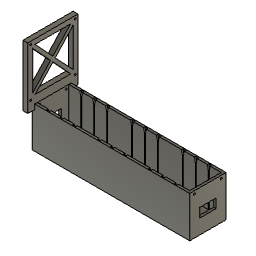
20220629_chipholder (Autodesk Fusion 360 design; units mm, degrees)
Autodesk Fusion 360 part; units mm, degrees
note: some values were not read from the file. Chosen so that the rebuilt part matches the saved one: a direction; which face or edge a step refers to. Set by a fixed rule: which sketch regions a step uses.
sketch "Sketch1" plane through (0, 0, 0) normal (0, 1, 0) x (1, 0, 0)
  line L0 (-25, -80) -> (231.8, -80) construction
  line L1 (0, 0) -> (0, -70.2552)
  line L2 (1.8, -70.2552) -> (1.8, 0)
  line L3 (0, -70.2552) -> (-2, -80)
  line L4 (1.8, -70.2552) -> (3.8, -80)
  line L5 (26.8, 0) -> (26.8, -70.2552)
  line L6 (28.6, -70.2552) -> (28.6, 0)
  line L7 (26.8, -70.2552) -> (24.8, -80)
  line L8 (28.6, -70.2552) -> (30.6, -80)
  line L9 (53.6, -70.2552) -> (53.6, 0)
  line L10 (160.8, 0) -> (160.8, -70.2552)
  line L11 (55.4, -70.2552) -> (55.4, 0)
  line L12 (105.4, 0) -> (105.4, -70.2552)
  line L13 (107.2, -70.2552) -> (107.2, 0)
  line L14 (132.2, 0) -> (132.2, -70.2552)
  line L15 (159, -70.2552) -> (159, 0)
  line L16 (212.6, 0) -> (212.6, -70.2552)
  line L17 (210.8, -70.2552) -> (210.8, 0)
  line L18 (134, 0) -> (134, -70.2552)
  line L19 (53.6, -70.2552) -> (51.6, -80)
  line L20 (55.4, -70.2552) -> (57.4, -80)
  line L21 (105.4, -70.2552) -> (103.4, -80)
  line L22 (132.2, -70.2552) -> (130.2, -80)
  line L23 (210.8, -70.2552) -> (208.8, -80)
  line L24 (212.6, -70.2552) -> (214.6, -80)
  line L25 (107.2, -70.2552) -> (109.2, -80)
  line L26 (134, -70.2552) -> (136, -80)
  line L27 (159, -70.2552) -> (157, -80)
  line L28 (160.8, -70.2552) -> (162.8, -80)
  line L29 (-25, -80) -> (291.2, -80)
  line L30 (291.2, 0) -> (-25, 0)
  line L31 (-25, 0) -> (-25, -80)
  line L32 (237.6, -70.2552) -> (237.6, 0)
  line L33 (239.4, 0) -> (239.4, -70.2552)
  line L34 (266.2, -70.2552) -> (266.2, 0)
  line L35 (264.4, -70.2552) -> (264.3999, 0)
  line L36 (237.6, -70.2552) -> (235.6, -80)
  line L37 (239.4, -70.2552) -> (241.4, -80)
  line L38 (264.4, -70.2552) -> (262.4, -80)
  line L39 (266.2, -70.2552) -> (268.2, -80)
  line L40 (291.2, 0) -> (291.2, -80)
  dimension "d5" = 1.8
  dimension "d6" = 2
  dimension "d7" = 2
  dimension "d8" = 25
  dimension "d9" = 1.8
  dimension "d10" = 2
  dimension "d11" = 2
  dimension "d12" = 25
  dimension "d13" = 1.8
  dimension "d14" = 50
  dimension "d15" = 1.8
  dimension "d16" = 25
  dimension "d17" = 1.8
  dimension "d18" = 25
  dimension "d19" = 1.8
  dimension "d20" = 50
  dimension "d21" = 1.8
  dimension "d22" = 2
  dimension "d23" = 2
  dimension "d24" = 2
  dimension "d25" = 2
  dimension "d26" = 2
  dimension "d27" = 2
  dimension "d28" = 2
  dimension "d29" = 2
  dimension "d30" = 2
  dimension "d31" = 2
  dimension "d89" = 25
  dimension "d90" = 1.8
  dimension "d91" = 25
  dimension "d92" = 1.8
  dimension "d93" = 2
  dimension "d94" = 2
  dimension "d95" = 2
  dimension "d96" = 2
  dimension "d97" = 25
  dimension "d98" = 25
  dimension "d99" = 80
  constraint coincident L0 L3.end
  constraint coincident L0 L4.end
  constraint coincident L0 L7.end
  constraint coincident L0 L8.end
  constraint coincident L0 L19.end
  constraint coincident L0 L20.end
  constraint midpoint L0 L21.end
  constraint coincident L0 L22.end
  constraint coincident L0 L23.end
  constraint coincident L0 L24.end
  constraint coincident L0 L25.end
  constraint coincident L0 L26.end
  constraint coincident L0 L27.end
  constraint coincident L0 L28.end
  constraint horizontal L29
  constraint horizontal L30
  constraint vertical L31
  constraint coincident L30 L32.end
  constraint coincident L30 L33.start
  constraint coincident L29 L36.end
  constraint coincident L29 L37.end
  constraint coincident L29 L38.end
  constraint coincident L29 L39.end
  constraint perpendicular L29 L40
  measures "d5" distance of L1 L2
  measures "d6" distance of L1 L3.end
  measures "d7" distance of L2 L4.end
  measures "d8" distance of L2 L5
  measures "d9" distance of L5 L6
  measures "d10" distance of L5 L7.end
  measures "d11" distance of L6 L8.end
  measures "d12" distance of L6 L9
  measures "d13" distance of L9 L11
  measures "d14" distance of L11 L12
  measures "d15" distance of L12 L13
  measures "d16" distance of L13 L14
  measures "d17" distance of L14 L18
  measures "d18" distance of L15 L18
  measures "d19" distance of L10 L15
  measures "d20" distance of L10 L17
  measures "d21" distance of L16 L17
  measures "d22" distance of L9 L19.end
  measures "d23" distance of L11 L20.end
  measures "d24" distance of L12 L21.end
  measures "d25" distance of L13 L25.end
  measures "d26" distance of L14 L22.end
  measures "d27" distance of L18 L26.end
  measures "d28" distance of L15 L27.end
  measures "d29" distance of L10 L28.end
  measures "d30" distance of L17 L23.end
  measures "d31" distance of L16 L24.end
  measures "d89" distance of L16 L32
  measures "d90" distance of L32 L33
  measures "d91" distance of L33 L35
  measures "d93" distance of L32 L36.end
  measures "d94" distance of L33 L37.end
  measures "d95" distance of L35 L38.end
  measures "d96" distance of L34 L39.end
  measures "d97" distance of L1 L31
  measures "d98" distance of L34 L40
  measures "d99" distance of L29 L30
extrude "Extrude1" add sketch "Sketch1" along normal blind 5 makes body 1
extrude "Extrude2" cut sketch "Sketch1" along normal blind 3 contours L1 L2 L3 L4 L29 L30 | L5 L6 L7 L8 L29 L30 | L9 L11 L19 L20 L29 L30 | L12 L13 L21 L25 L29 L30 | L14 L18 L22 L26 L29 L30 | L10 L15 L27 L28 L29 L30 | L16 L17 L23 L24 L29 L30 bodies 1
sketch "Sketch1 (2)" plane through (0, 0, 0) normal (0, 0, 1) x (1, 0, 0) in component "carrier"
  line L0 (-40.0005, -7.3553) -> (29.9995, -7.3553)
  line L1 (29.9995, -7.3553) -> (29.9995, 62.6447)
  line L2 (-40.0005, 62.6447) -> (-40.0005, -7.3553)
  line L3 (-40.0005, 62.6447) -> (-31.0005, 62.6447)
  line L4 (29.9995, 62.6447) -> (20.9995, 62.6447)
  line L5 (-31.0005, 62.6447) -> (-31.0005, 79.6447)
  line L6 (20.9995, 62.6447) -> (20.9995, 79.6447)
  line L7 (20.9995, 79.6447) -> (44.9995, 79.6447)
  line L8 (44.9995, 79.6447) -> (44.9995, 187.4447)
  line L9 (44.9995, 187.4447) -> (-55.0005, 187.4447)
  line L10 (-55.0005, 187.4447) -> (-55.0005, 79.6447)
  line L11 (-55.0005, 79.6447) -> (-31.0005, 79.6447)
  circle A0 centre (-51.1505, 83.4947) radius 1.95
  circle A1 centre (41.1495, 83.4947) radius 1.95
  circle A2 centre (41.1495, 183.5947) radius 1.95
  circle A3 centre (-51.1505, 183.5947) radius 1.95
  line L12 (75.2881, -7.3553) -> (70.2881, -7.3553)
  dimension "d18_1" = 70
  dimension "d23_1" = 9
  dimension "d24_1_1" = 9
  dimension "d25_1_1" = 70
  dimension "d26_1_1" = 52
  dimension "d27_1_1" = 17
  dimension "d28_1" = 17
  dimension "d29_1_1" = 70
  dimension "d47" = 107.8
  dimension "d48" = 100
  dimension "d49" = 3.9
  dimension "d50" = 3.85
  dimension "d51" = 3.85
  dimension "d52" = 3.9
  dimension "d53" = 3.9
  dimension "d54" = 3.9
  dimension "d55" = 3.85
  dimension "d56" = 3.85
  dimension "d57" = 3.85
  dimension "d58" = 3.85
  dimension "d59" = 3.85
  dimension "d60" = 3.85
  constraint horizontal L0
  constraint vertical L1
  constraint vertical L2
  constraint perpendicular L1 L4
  constraint perpendicular L6 L7
  constraint perpendicular L7 L8
  constraint perpendicular L8 L9
  constraint perpendicular L9 L10
  constraint perpendicular L5 L11
  constraint equal L7 L11
  constraint collinear L0 L12
  constraint parallel L0 L9
  measures "d18_1" distance of L0.start L0.end
  measures "d23_1" distance of L2.start L3.end
  measures "d24_1_1" distance of L1.end L4.end
  measures "d25_1_1" distance of L0.end L1.end
  measures "d26_1_1" distance of L5.end L6.end
  measures "d27_1_1" distance of L4.end L6.end
  measures "d28_1" distance of L3.end L5.end
  measures "d29_1_1" distance of L0.start L2.start
  measures "d47" distance of L9 L11
  measures "d48" distance of L8 L10
  measures "d49" diameter of A0
  measures "d50" distance of L11 A0.centre
  measures "d51" distance of L10 A0.centre
  measures "d52" diameter of A1
  measures "d53" diameter of A2
  measures "d54" diameter of A3
  measures "d55" distance of L7 A1.centre
  measures "d56" distance of L8 A1.centre
  measures "d57" distance of L9 A3.centre
  measures "d58" distance of L10 A3.centre
  measures "d59" distance of L9 A2.centre
  measures "d60" distance of L8 A2.centre
extrude "Extrude1'" add sketch "Sketch1 (2)" along normal blind 1.6 separate body contours L0 L1 L2 L3 L4 L5 L6 L7 L8 L9 L10 L11 | A0 | A1 | A2 | A3 makes body 2 in component "carrier"
sketch "Sketch2" plane through (0, 0, 1.7) normal (0, 0, 1) x (-1, 0, 0) in component "carrier"
  line L0 (-200, -70) -> (-200, 0)
  line L1 (-200, 0) -> (-270, 0)
  line L2 (-270, 0) -> (-270, -70)
  line L3 (-270, -70) -> (-261, -70)
  line L4 (-261, -70) -> (-261, -83.4)
  line L5 (-261, -83.4) -> (-209, -83.4)
  line L6 (-209, -83.4) -> (-209, -70)
  line L7 (-209, -70) -> (-200, -70)
  line L8 (-207, -21) -> (-207, -49)
  line L9 (-270, 0) -> (-268.2738, 0)
  line L10 (-268.2738, -21) -> (-270, -21)
  line L11 (-270, -21) -> (-268.2738, -21)
  line L12 (-263, -21) -> (-263, -49)
  line L13 (-207, -49) -> (-263, -49)
  line L14 (-207, -21) -> (-263, -21)
  dimension "d38_1" = 7
  dimension "d39_1_1" = 7
  dimension "d40_1_1" = 21
  dimension "d41_1_1" = 21
  constraint horizontal L9
  constraint horizontal L10
  constraint coincident L1.end L2.start
  constraint perpendicular L2 L11
  constraint perpendicular L11 L12
  measures "d38_1" distance of L0 L8
  measures "d39_1_1" distance of L2 L12
  measures "d40_1_1" distance of L1 L14
  measures "d41_1_1" distance of L3 L13
extrude "Extrude2'" [suppressed] in component "carrier"
sketch "Sketch3" plane through (0, 0, 6.2) normal (0, 0, 1) x (-1, 0, 0) in component "carrier"
  line L0 (-207, -49) -> (-207, -21)
  line L1 (-207, -21) -> (-263, -21)
  line L2 (-263, -21) -> (-263, -49)
  line L3 (-263, -49) -> (-207, -49)
  circle A0 centre (-209.7, -35) radius 2.7
  line L4 (-270, 0) -> (-235, 0) construction
  line L5 (-235, 0) -> (-235, -95) construction
  circle A1 centre (-260.3, -35) radius 2.7
  dimension "d44_1_1" = 5.4
  dimension "d45_1" = 14
  dimension "d47_1" = 2.7
  dimension "d48_1" = 35
  dimension "d49_1" = 14
  dimension "d50_1" = 2.7
  constraint horizontal L4
  constraint perpendicular L1 L5
  constraint symmetric A0 L5 A1
  measures "d44_1_1" diameter of A0
  measures "d45_1" distance of L1 A0.centre
  measures "d47_1" distance of L0 A0.centre
  measures "d48_1" distance of L4.start L4.end
  measures "d49_1" distance of L3 A1.centre
  measures "d50_1" distance of L2 A1.centre
extrude "Extrude4" [suppressed] in component "carrier"
extrude "Extrude3" [suppressed] in component "carrier"
sketch "Sketch5" plane through (0, 0, 0) normal (0, 0, -1) x (1, 0, 0) in component "carrier"
  line L0 (200, 0) -> (200, -70)
  line L1 (200, -70) -> (209, -70)
  line L2 (209, -70) -> (209, -83.4)
  line L3 (209, -83.4) -> (261, -83.4)
  line L4 (261, -83.4) -> (261, -70)
  line L5 (261, -70) -> (270, -70)
  line L6 (270, -70) -> (270, 0)
  line L7 (270, 0) -> (200, 0)
  line L8 (206.7865, -21) -> (206.7865, -49)
  line L9 (263, -21) -> (263, -49)
  line L10 (206.7865, -21) -> (263, -21)
  line L11 (206.7865, -49) -> (263, -49)
  dimension "d61_1" = 28
  dimension "d62_1" = 28
  constraint perpendicular L9 L10
  constraint perpendicular L9 L11
  measures "d61_1" distance of L8.start L8.end
  measures "d62_1" distance of L9.start L9.end
extrude "Extrude6" [suppressed] in component "carrier"
sketch "Sketch7" plane through (0, 0, -4.5) normal (0, 0, -1) x (1, 0, 0) in component "carrier"
  line L0 (206.7865, -21) -> (206.7865, -49)
  line L1 (206.7865, -49) -> (263, -49)
  line L2 (263, -49) -> (263, -21)
  line L3 (263, -21) -> (206.7865, -21)
  circle A0 centre (209.4865, -35) radius 2.7
  line L4 (206.7865, -21) -> (206.7865, -49)
  line L5 (206.7865, -21) -> (263, -21)
  line L6 (235, 0) -> (235, -95)
  circle A1 centre (260.5135, -35) radius 2.7
  dimension "d73_1" = 5.4
  dimension "d74_1" = 2.7
  dimension "d75_1" = 14
  constraint symmetric A0 L6 A1
  measures "d73_1" diameter of A0
  measures "d74_1" distance of A0.centre L4
  measures "d75_1" distance of A0.centre L5
extrude "Extrude8" [suppressed] in component "carrier"
extrude "Extrude7" [suppressed] in component "carrier"
sketch "Sketch8" plane through (0, 0, -6.8) normal (0, 0, -1) x (1, 0, 0) in component "carrier"
  circle A0 centre (209.4865, -35) radius 2.7
  circle A1 centre (209.4865, -35) radius 1.5
  dimension "d80_1" = 3
  constraint concentric A0 A1
  measures "d80_1" diameter of A1
extrude "Extrude9" [suppressed] in component "carrier"
sketch "Sketch10" plane through (0, 0, -6.8) normal (0, 0, -1) x (1, 0, 0) in component "carrier"
  line L0 (263, -36.0522) -> (263, -33.9478)
  arc A0 (263, -33.9478) -> (263, -36.0522) centre (260.5135, -35) ccw
  circle A1 centre (260.5135, -35) radius 1.5
  dimension "d84_1" = 3
  constraint concentric A0 A1
  measures "d84_1" diameter of A1
extrude "Extrude10" [suppressed] in component "carrier"
sketch "Sketch1 (3)" plane through (0, 0, 1.6) normal (0, 0, 1) x (-1, 0, 0) in component "alpide sensor"
  circle A0 centre (-65, -5) radius 1.5
  circle A1 centre (-5, -5) radius 1.5
  circle A2 centre (-65, -65) radius 1.5
  circle A3 centre (-5, -65) radius 1.5
  line L0 (0, -70) -> (0, 0)
  line L1 (0, 0) -> (-70, 0)
  line L2 (-70, 0) -> (-70, -70)
  line L3 (-70, -70) -> (-61, -70)
  line L4 (-61, -70) -> (-61, -83.5)
  line L5 (-61, -83.5) -> (-9, -83.5)
  line L6 (-9, -83.5) -> (-9, -70)
  line L7 (-9, -70) -> (0, -70)
  line L8 (-20, -42.5) -> (-50, -42.5)
  line L9 (-50, -42.5) -> (-50, -27.5)
  line L10 (-50, -27.5) -> (-20, -27.5)
  line L11 (-20, -27.5) -> (-20, -42.5)
  dimension "d58_1" = 30
  dimension "d59_1" = 15
  dimension "d60_1" = 41
  dimension "d63_1" = 20
  constraint horizontal L8
  constraint vertical L9
  constraint horizontal L10
  constraint vertical L11
  measures "d58_1" distance of L8.start L8.end
  measures "d59_1" distance of L8.start L10.end
  measures "d60_1" distance of L5 L8
  measures "d63_1" distance of L2 L9
extrude "Extrude1''" add sketch "Sketch1 (3)" along normal blind -1.8 and the other way blind -0.1 separate body contours L8 L9 L10 L11 makes body 3 in component "alpide sensor"
extrude "Extrude11" cut sketch "Sketch1 (2)" along normal blind 5 contours A0 | A1 | A2 | A3 bodies 2 in component "carrier"
move_body "Move1" bodies 2 to x (1, 0, 0) y (0, 1, 0) z (0, 0, 1) at (42.3005, 7.3553, 24.9) in component "carrier"
move_body "Move2" bodies 2 to x (1, 0, 0) y (0, 1, 0) z (0, 0, 1) at (-3, 0, 0) in component "carrier"
move_body "Move3" bodies 2 to x (1, 0, 0) y (0, 1, 0) z (0, 0, 1) at (0.7, 0, 0.1) in component "carrier"
sketch "Sketch4" plane through (-25, 0, 0) normal (-1, 0, 0) x (0, -1, 0)
  line L0 (0, 0) -> (0, 80)
  line L1 (0, 80) -> (-5, 80)
  line L2 (-5, 80) -> (-5, 0)
  line L3 (-5, 0) -> (0, 0)
  line L4 (-5, 80) -> (0, 80)
  line L5 (70.4, 80) -> (70.4, -5)
  line L6 (70.4, -5) -> (-5, -5)
  line L7 (-5, -5) -> (-5, 80)
  line L8 (70.4, 80) -> (70.4, 0)
  line L9 (70.4, -5) -> (-5, -5)
  line L10 (65.4, 80) -> (70.4, 80)
  line L11 (17.7, 42.5) -> (47.7, 42.5)
  line L12 (47.7, 42.5) -> (47.7, 27.5)
  line L13 (47.7, 27.5) -> (17.7, 27.5)
  line L14 (17.7, 27.5) -> (17.7, 42.5)
  line L15 (17.7, 42.5) -> (17.7, 27.5)
  line L16 (47.7, 42.5) -> (17.7, 42.5)
  line L17 (47.7, 27.5) -> (47.7, 42.5)
  line L18 (17.7, 27.5) -> (47.7, 27.5)
  line L19 (15.7, 44.5) -> (49.7, 44.5)
  line L20 (49.7, 44.5) -> (49.7, 25.5)
  line L21 (49.7, 25.5) -> (15.7, 25.5)
  line L22 (15.7, 25.5) -> (15.7, 44.5)
  line L23 (-19.3, 196.8) -> (84.7, 196.8)
  line L24 (84.7, 196.8) -> (84.7, 80)
  line L25 (-19.3, 80) -> (-19.3, 196.8)
  line L26 (82.7, 194.8) -> (-17.3, 194.8)
  line L27 (82.7, 87) -> (82.7, 194.8)
  line L28 (-17.3, 194.8) -> (-17.3, 87)
  circle A0 centre (78.85, 90.85) radius 1.95
  circle A1 centre (78.85, 90.85) radius 1.95
  circle A2 centre (78.85, 190.95) radius 1.95
  circle A3 centre (78.85, 190.95) radius 1.95
  circle A4 centre (-13.45, 190.95) radius 1.95
  circle A5 centre (-13.45, 190.95) radius 1.95
  circle A6 centre (-13.45, 90.85) radius 1.95
  circle A7 centre (-13.45, 90.85) radius 1.95
  line L29 (84.7, 80) -> (70.4, 80)
  line L30 (0, 80) -> (-19.3, 80)
  line L31 (-9.3, 186.8) -> (74.7, 186.8)
  line L32 (74.7, 186.8) -> (74.7, 96.85)
  line L33 (74.7, 96.85) -> (-9.3, 96.85)
  line L34 (-9.3, 96.85) -> (-9.3, 186.8)
  line L35 (-9.3, 100.85) -> (28.8385, 141.825)
  line L36 (32.7, 145.9737) -> (70.7, 186.8)
  line L37 (74.7, 182.8) -> (36.5615, 141.825)
  line L38 (32.7, 137.6762) -> (-5.3, 96.85)
  line L39 (74.7, 100.85) -> (36.5615, 141.825)
  line L40 (32.7, 145.9737) -> (-5.3, 186.8)
  line L41 (-9.3, 182.8) -> (28.8385, 141.825)
  line L42 (32.7, 137.6762) -> (70.7, 96.85)
  point P0 (-5, 80)
  dimension "d63" = 2
  dimension "d64" = 2
  dimension "d65" = 2
  dimension "d66" = 2
  dimension "d68" = 2
  dimension "d69" = 2
  dimension "d70" = 2
  dimension "d71" = 3.9
  dimension "d72" = 3.9
  dimension "d73" = 3.9
  dimension "d74" = 3.9
  dimension "d75" = 10
  dimension "d76" = 10
  dimension "d77" = 10
  dimension "d78" = 6
  dimension "d79" = 4
  dimension "d80" = 4
  dimension "d81" = 4
  dimension "d82" = 4
  dimension "d83" = 4
  dimension "d84" = 4
  dimension "d85" = 4
  dimension "d86" = 4
  constraint horizontal L4
  constraint vertical L5
  constraint horizontal L6
  constraint vertical L7
  constraint collinear L5 L8
  constraint collinear L6 L9
  constraint collinear L2 L7
  constraint collinear L4 L10
  constraint horizontal L11
  constraint vertical L12
  constraint horizontal L13
  constraint vertical L14
  constraint collinear L14 L15
  constraint collinear L11 L16
  constraint collinear L12 L17
  constraint collinear L13 L18
  constraint horizontal L19
  constraint vertical L20
  constraint horizontal L21
  constraint vertical L22
  constraint horizontal L23
  constraint vertical L24
  constraint horizontal L29
  constraint vertical L25
  constraint coincident P0 L29
  constraint concentric A0 A1
  constraint concentric A2 A3
  constraint concentric A4 A5
  constraint concentric A6 A7
  constraint collinear L29 L30
  constraint horizontal L31
  constraint vertical L32
  constraint horizontal L33
  constraint vertical L34
  constraint coincident L34 L35.start
  constraint coincident L31 L36.end
  constraint coincident L32 L37.start
  constraint coincident L33 L38.end
  constraint coincident L34 L41.start
  constraint coincident L33 L42.end
  constraint coincident L32 L39.start
  constraint coincident L31 L40.end
  constraint coincident L36.start L39
  constraint collinear L35 L36
  constraint coincident L38.start L41
  constraint collinear L37 L38
  constraint collinear L39 L40
  constraint collinear L41 L42
  measures "d63" distance of L11 L19
  measures "d64" distance of L12 L20
  measures "d65" distance of L13 L21
  measures "d66" distance of L14 L22
  measures "d68" distance of L23 L26
  measures "d69" distance of L24 L27
  measures "d70" distance of L25 L28
  measures "d71" diameter of A0
  measures "d72" diameter of A2
  measures "d73" diameter of A4
  measures "d74" diameter of A6
  measures "d75" distance of L25 L34
  measures "d76" distance of L23 L31
  measures "d77" distance of L24 L32
  measures "d78" distance of A6.centre L33
  measures "d79" distance of L33.end L35.start
  measures "d80" distance of L31.end L36.end
  measures "d81" distance of L33.end L38.end
  measures "d82" distance of L31.end L37.start
  measures "d83" distance of L31.start L40.end
  measures "d84" distance of L31.start L41.start
  measures "d85" distance of L32.end L39.start
  measures "d86" distance of L32.end L42.end
extrude "Extrude6'" cut sketch "Sketch1" along normal blind 3 contours L29 L30 L32 L33 L36 L37 bodies 1
extrude "Extrude7'" cut sketch "Sketch1" along normal blind 3 contours L29 L30 L34 L35 L38 L39 bodies 1
move_body "Move9" bodies 1 to x (1, 0, 0) y (0, 1, 0) z (0, 0, 1) at (25, 0, 0)
copy_body "CopyPasteBodies3" bodies 1 makes body 4
move_body "Move10" bodies 4 to x (1, 0, 0) y (0, 1, 0) z (0, 0, 1) at (0, -70.4, 0)
move_body "Move11" bodies 4 to x (-1, 0, 0) y (0, -1, 0) z (0, 0, 1) at (314.4, -140.8, 0)
move_body "Move12" bodies 4 to x (1, 0, 0) y (0, 1, 0) z (0, 0, 1) at (1.8, 5, 0)
sketch "Sketch5 (2)" plane through (0, 0, 0) normal (0, 0, -1) x (1, 0, 0)
  line L0 (26.8001, 68.4) -> (26.8001, 65.4)
  line L1 (26.8001, 65.4) -> (51.8, 65.4)
  line L2 (51.8, 65.4) -> (51.8, 68.4)
  line L3 (51.8, 68.4) -> (53.6, 68.4)
  line L4 (53.6, 68.4) -> (53.6, 65.4)
  line L5 (53.6, 65.4) -> (78.6, 65.4)
  line L6 (78.6, 65.4) -> (78.6, 68.4)
  line L7 (78.6, 68.4) -> (80.4, 68.4)
  line L8 (80.4, 68.4) -> (80.4, 65.4)
  line L9 (80.4, 65.4) -> (130.4, 65.4)
  line L10 (130.4, 65.4) -> (130.4, 68.4)
  line L11 (130.4, 68.4) -> (132.2, 68.4)
  line L12 (132.2, 68.4) -> (132.2, 65.4)
  line L13 (132.2, 65.4) -> (157.2, 65.4)
  line L14 (157.2, 65.4) -> (157.2, 68.4)
  line L15 (157.2, 68.4) -> (159, 68.4)
  line L16 (159, 68.4) -> (159, 65.4)
  line L17 (159, 65.4) -> (184, 65.4)
  line L18 (184, 65.4) -> (184, 68.4)
  line L19 (184, 68.4) -> (185.8, 68.4)
  line L20 (185.8, 68.4) -> (185.8, 65.4)
  line L21 (185.8, 65.4) -> (235.8, 65.4)
  line L22 (235.8, 65.4) -> (235.8, 68.4)
  line L23 (235.8, 68.4) -> (237.6, 68.4)
  line L24 (237.6, 68.4) -> (237.6, 65.4)
  line L25 (237.6, 65.4) -> (262.6, 65.4)
  line L26 (262.6, 65.4) -> (262.6, 68.4)
  line L27 (262.6, 68.4) -> (264.4, 68.4)
  line L28 (264.4, 68.4) -> (264.4, 65.4)
  line L29 (264.4, 65.4) -> (289.4, 65.4)
  line L30 (289.4, 65.4) -> (289.4, 68.4)
  line L31 (289.4, 68.4) -> (291.2, 68.4)
  line L32 (291.2, 68.4) -> (291.2, 65.4)
  line L33 (291.2, 65.4) -> (316.2, 65.4)
  line L34 (316.2, 65.4) -> (316.2, 70.4)
  line L35 (316.2, 70.4) -> (0, 70.4)
  line L36 (0, 70.4) -> (0, 65.4)
  line L37 (0, 65.4) -> (25, 65.4)
  line L38 (25, 65.4) -> (25, 68.4)
  line L39 (25, 68.4) -> (26.8001, 68.4)
  line L40 (0, 70.4) -> (316.2, 70.4)
  line L41 (316.2, 70.4) -> (316.2, -5)
  line L42 (316.2, -5) -> (0, -5)
  line L43 (0, -5) -> (0, 70.4)
  line L44 (316.2, -5) -> (0, -5)
  constraint horizontal L40
  constraint vertical L41
  constraint horizontal L42
  constraint vertical L43
  constraint collinear L35 L40
  constraint collinear L36 L43
  constraint collinear L34 L41
  constraint collinear L42 L44
extrude "Extrude8'" add sketch "Sketch5 (2)" along normal blind 5 separate body makes body 5
move_body "Move4" bodies 2 to x (1, 0, 0) y (0, 1, 0) z (0, 0, 1) at (0.7, 0, -25.1001) in component "carrier"
move_body "Move5" bodies 2 to x (1, 0, 0) y (0, 1, 0) z (0, 0, 1) at (-0.7, 0, 0.1) in component "carrier"
move_body "Move6" bodies 2 to x (1, 0, 0) y (0, 1, 0) z (0, 0, 1) at (0.7, 0, -0.1) in component "carrier"
move_body "Move7" bodies 2 to x (1, 0, 0) y (0, 1, 0) z (0, 0, 1) at (-0.7, 0, 0) in component "carrier"
move_body "Move8" bodies 2 to x (1, 0, 0) y (0, 1, 0) z (0, 0, 1) at (0, 0, 0.1) in component "carrier"
sketch "Sketch6" plane through (0, 0, 0) normal (-1, 0, 0) x (0, -1, 0)
  line L0 (0, 0) -> (0, 80)
  line L1 (0, 80) -> (-5, 80)
  line L2 (-5, 80) -> (-5, 0)
  line L3 (-5, 0) -> (0, 0)
  line L4 (-5, 80) -> (70.4, 80)
  line L5 (70.4, 80) -> (70.4, -5)
  line L6 (70.4, -5) -> (-5, -5)
  line L7 (-5, -5) -> (-5, 80)
  line L8 (70.4, 80) -> (70.4, 0)
  line L9 (70.4, -5) -> (-5, -5)
  line L10 (17.7, 42.5) -> (47.7, 42.5)
  line L11 (47.7, 42.5) -> (47.7, 27.5)
  line L12 (47.7, 27.5) -> (17.7, 27.5)
  line L13 (17.7, 27.5) -> (17.7, 42.5)
  line L14 (47.7, 42.5) -> (17.7, 42.5)
  line L15 (17.7, 42.5) -> (17.7, 27.5)
  line L16 (17.7, 27.5) -> (47.7, 27.5)
  line L17 (47.7, 27.5) -> (47.7, 42.5)
  line L18 (15.7, 44.5) -> (49.7, 44.5)
  line L19 (49.7, 44.5) -> (49.7, 25.5)
  line L20 (49.7, 25.5) -> (15.7, 25.5)
  line L21 (15.7, 25.5) -> (15.7, 44.5)
  circle A0 centre (5, 74) radius 1.95
  circle A1 centre (60.4, 74) radius 1.95
  dimension "d107" = 2
  dimension "d108" = 2
  dimension "d109" = 2
  dimension "d110" = 2
  dimension "d115" = 3.9
  dimension "d116" = 3.9
  dimension "d117" = 10
  dimension "d118" = 10
  dimension "d119" = 6
  dimension "d120" = 6
  constraint horizontal L4
  constraint vertical L5
  constraint horizontal L6
  constraint vertical L7
  constraint collinear L1 L4
  constraint collinear L2 L7
  constraint collinear L5 L8
  constraint collinear L6 L9
  constraint horizontal L10
  constraint vertical L11
  constraint horizontal L12
  constraint vertical L13
  constraint collinear L10 L14
  constraint collinear L13 L15
  constraint collinear L12 L16
  constraint collinear L11 L17
  constraint horizontal L18
  constraint vertical L19
  constraint horizontal L20
  constraint vertical L21
  measures "d107" distance of L10 L18
  measures "d108" distance of L13 L21
  measures "d109" distance of L12 L20
  measures "d110" distance of L11 L19
  measures "d115" diameter of A0
  measures "d116" diameter of A1
  measures "d117" distance of L7 A0.centre
  measures "d118" distance of L5 A1.centre
  measures "d119" distance of L4 A0.centre
  measures "d120" distance of L4 A1.centre
extrude "Extrude9'" add sketch "Sketch6" along normal blind 5 separate body contours L0 L1 L2 L3 L4 L7 | L0 L3 L4 L5 L6 L7 L8 L9 | A0 | A1 makes body 6
extrude "Extrude10'" cut sketch "Sketch6" along normal blind 5 contours A0 | A1 bodies 6
sketch "Sketch9" plane through (-5, 0, 0) normal (-1, 0, 0) x (0, -1, 0)
  circle A0 centre (60.4, 74) radius 1.95
  circle A1 centre (5, 74) radius 1.95
  line L0 (49.7, 25.5) -> (15.7, 25.5)
  line L1 (15.7, 25.5) -> (15.7, 44.5)
  line L2 (15.7, 44.5) -> (49.7, 44.5)
  line L3 (49.7, 44.5) -> (49.7, 25.5)
  line L4 (70.4, -5) -> (70.4, 80)
  line L5 (70.4, 80) -> (-5, 80)
  line L6 (-5, 80) -> (-5, -5)
  line L7 (-5, -5) -> (70.4, -5)
  line L8 (82.7, 194.8) -> (-17.3, 194.8)
  line L9 (-17.3, 194.8) -> (-17.3, 87)
  line L10 (82.7, 87) -> (82.7, 194.8)
  line L11 (-5, 80) -> (70.4, 80)
  circle A2 centre (-13.45, 90.85) radius 1.95
  circle A3 centre (-13.45, 90.85) radius 1.95
  circle A4 centre (78.85, 90.85) radius 1.95
  circle A5 centre (78.85, 190.95) radius 1.95
  circle A6 centre (-13.45, 190.95) radius 1.95
  circle A7 centre (-13.45, 190.95) radius 1.95
  circle A8 centre (78.85, 190.95) radius 1.95
  circle A9 centre (78.85, 90.85) radius 1.95
  circle A10 centre (5, 74) radius 1.95
  circle A11 centre (60.4, 74) radius 1.95
  circle A12 centre (5, 74) radius 1.95
  circle A13 centre (60.4, 74) radius 1.95
  line L12 (84.7, 196.8) -> (-19.3, 196.8)
  line L13 (-19.3, 196.8) -> (-19.3, 70)
  line L14 (-19.3, 70) -> (84.7, 70)
  line L15 (84.7, 70) -> (84.7, 196.8)
  line L16 (-9.3, 186.8) -> (74.7, 186.8)
  line L17 (74.7, 186.8) -> (74.7, 96.85)
  line L18 (74.7, 96.85) -> (-9.3, 96.85)
  line L19 (-9.3, 96.85) -> (-9.3, 186.8)
  line L20 (-9.3, 101.85) -> (69.7, 186.8)
  line L21 (74.7, 181.8) -> (-4.3, 96.85)
  line L22 (-9.3, 181.8) -> (69.7, 96.85)
  line L23 (-4.3, 186.8) -> (74.7, 101.85)
  dimension "d124" = 3.9
  dimension "d125" = 3.9
  dimension "d126" = 3.9
  dimension "d127" = 3.9
  dimension "d128" = 3.9
  dimension "d129" = 3.9
  dimension "d130" = 2
  dimension "d131" = 2
  dimension "d132" = 2
  dimension "d133" = 10
  dimension "d134" = 10
  dimension "d135" = 10
  dimension "d136" = 6
  dimension "d137" = 10
  dimension "d138" = 5
  dimension "d139" = 5
  dimension "d140" = 5
  dimension "d141" = 5
  dimension "d142" = 5
  dimension "d143" = 5
  dimension "d144" = 5
  dimension "d145" = 5
  constraint concentric A2 A3
  constraint concentric A6 A7
  constraint concentric A5 A8
  constraint concentric A4 A9
  constraint concentric A10 A12
  constraint concentric A11 A13
  constraint horizontal L12
  constraint vertical L13
  constraint horizontal L14
  constraint vertical L15
  constraint horizontal L16
  constraint vertical L17
  constraint horizontal L18
  constraint vertical L19
  constraint coincident L19 L20.start
  constraint coincident L16 L20.end
  constraint coincident L17 L21.start
  constraint coincident L18 L21.end
  constraint coincident L19 L22.start
  constraint coincident L18 L22.end
  constraint coincident L16 L23.start
  constraint coincident L17 L23.end
  measures "d124" diameter of A2
  measures "d125" diameter of A4
  measures "d126" diameter of A5
  measures "d127" diameter of A6
  measures "d128" diameter of A10
  measures "d129" diameter of A11
  measures "d130" distance of L8 L12
  measures "d131" distance of L10 L15
  measures "d132" distance of L9 L13
  measures "d133" distance of L11 L14
  measures "d134" distance of L12 L16
  measures "d135" distance of L15 L17
  measures "d136" distance of A4.centre L18
  measures "d137" distance of L13 L19
  measures "d138" distance of L16.start L22.start
  measures "d139" distance of L16.start L23.start
  measures "d140" distance of L16.end L20.end
  measures "d141" distance of L16.end L21.start
  measures "d142" distance of L17.end L23.end
  measures "d143" distance of L17.end L22.end
  measures "d144" distance of L18.end L21.end
  measures "d145" distance of L18.end L20.start
extrude "Extrude11'" add sketch "Sketch9" along normal blind 5 separate body contours L4 L5 L6 L11 L14 | L4 L5 L6 L11 L12 L13 L14 L15 | L16 L19 L20 L22 L23 | L16 L17 L20 L21 L23 | L20 L21 L22 L23 | L18 L19 L20 L21 L22 | L17 L18 L21 L22 L23 makes body 7
extrude "Extrude12" add sketch "Sketch9" against normal blind 5 separate body contours L4 L5 L6 L11 L12 L13 L14 L15 | L16 L19 L20 L22 L23 | L16 L17 L20 L21 L23 | L20 L21 L22 L23 | L18 L19 L20 L21 L22 | L17 L18 L21 L22 L23 makes body 8
combine "Combine1" operation add target body 8 tool bodies 7
extrude "Extrude14" cut sketch "Sketch9" against normal blind 5 contours A0 A11 A13 | A1 A10 A12 bodies 6
copy_body "CopyPasteBodies5" bodies 8 6 makes body 9 makes body 10
move_body "Move16" bodies 9 10 to x (-1, 0, 0) y (0, -1, 0) z (0, 0, 1) at (-20, -169.4, 0)
move_body "Move17" bodies 9 10 to x (1, 0, 0) y (0, 1, 0) z (0, 0, 1) at (336.2, 104, 0)
combine "Combine2" operation add target body 10 tool bodies 6 5 4 1
component "carrier chip v5" placed x (0, -1, 0) y (0, 0, 1) z (-1, 0, 0) at (45.4, 73.6, 4.0098)
component "carrier" placed x (1, 0, 0) y (0, 1, 0) z (0, 0, 1) at (71.3, -4.0098, 18.7) in component "carrier chip v5"
component "alpide sensor" placed x (1, 0, 0) y (0, 1, 0) z (0, 0, 1) at (0, 0, 0) in component "carrier"
hidden bodies 9
equation "d7 = d6"
equation "d9 = d5"
equation "d10 = d6"
equation "d11 = d6"
equation "d12 = d8"
equation "d13 = d5"
equation "d15 = d5"
equation "d16 = d8"
equation "d17 = d5"
equation "d18 = d8"
equation "d19 = d5"
equation "d20 = d14"
equation "d21 = d5"
equation "d22 = d6"
equation "d23 = d6"
equation "d24 = d6"
equation "d25 = d6"
equation "d26 = d6"
equation "d27 = d6"
equation "d28 = d6"
equation "d29 = d6"
equation "d30 = d6"
equation "d31 = d6"
equation "d27_1_1 = d28_1"
equation "d50 = 1.9 mm + ( 3.9 / 2 ) * 1 mm"
equation "d51 = 1.9 mm + ( 3.9 / 2 ) * 1 mm"
equation "d55 = d50"
equation "d56 = d51"
equation "d57 = d50"
equation "d58 = d51"
equation "d59 = d57"
equation "d60 = d58"
equation "d76 = d75"
equation "d77 = d76"
equation "d78 = 4 mm + 2 mm"
equation "d81 = d79"
equation "d86 = d85"
equation "d89 = d8"
equation "d90 = d5"
equation "d91 = d8"
equation "d92 = d5"
equation "d93 = d6"
equation "d94 = d6"
equation "d95 = d6"
equation "d96 = d6"
equation "d97 = d8"
equation "d98 = d8"
equation "d108 = d107"
equation "d109 = d107"
equation "d110 = d107"
equation "d118 = d117"
equation "d120 = d119"
equation "d124 = d125"
equation "d126 = d125"
equation "d127 = d126"
equation "d128 = d125"
equation "d129 = d125"
equation "d139 = d138"
equation "d140 = d138"
equation "d141 = d138"
equation "d142 = d138"
equation "d143 = d138"
equation "d144 = d138"
equation "d145 = d138"
